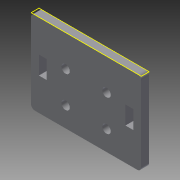
# Autodesk Inventor part: hook faceplate
Saved by Autodesk Inventor 2013 (Build 170138000, 138)
## iProperties
Created: 2013-01-26
Part Number: hook faceplate
Material: Generic
Document SubType Name: Modeling
Designer: Arpan
Density: 1 g/cm^3
Mass: 36.5886 g
Surface Area: 140.029 cm^2
Volume: 36.5886 cm^3
Author: Arpan
Autodesk Inventor part; units mm, degrees
ref_plane "YZ Plane" through (0, 0, 0) normal (1, 0, 0) x (0, 1, 0)
ref_plane "XZ Plane" through (0, 0, 0) normal (0, 1, 0) x (-1, 0, 0)
ref_plane "XY Plane" through (0, 0, 0) normal (0, 0, 1) x (1, 0, 0)
sketch "Sketch1" plane through (0, 0, 0) normal (0, 0, 1) x (1, 0, 0)
  line L0 (0, 0) -> (-88.9, 0)
  line L1 (-88.9, 0) -> (-88.9, 67.0052)
  line L2 (-88.9, 67.0052) -> (0, 67.0052)
  line L3 (0, 67.0052) -> (0, 0)
  dimension "d0" = 88.9
  dimension "d1" = 67.0052
  dimension "d2" = 90
  constraints: 8 end point, 2 perpendicular, 1 horizontal
  measures "d0" distance of L0.start L0.end
  measures "d1" distance of L0.end L1.end
  measures "d2" angle of L0 L3
extrude "Extrusion1" add sketch "Sketch1" along normal blind 6.35
sketch "Sketch2" plane through (-88.9, 67.0052, 0) normal (0, 1, 0) x (1, 0, 0)
  line L0 (0, 0) -> (88.9, 0) projected
  line L1 (0, 0) -> (0, -6.35) projected
  line L2 (88.9, -6.35) -> (0, -6.35) projected
  line L3 (88.9, 0) -> (88.9, -6.35) projected
sketch "Sketch3" plane through (0, 0, 0) normal (0, 0, -1) x (-1, 0, 0)
  line L0 (88.9, 0) -> (88.9, 67.0052) projected
  line L1 (0, 67.0052) -> (0, 0) projected
  line L2 (0, 67.0052) -> (0, 40.8178)
  line L3 (0, 40.8178) -> (6.35, 40.8178)
  line L4 (6.35, 40.8178) -> (6.35, 26.162)
  line L5 (6.35, 26.162) -> (12.7, 26.162)
  line L6 (12.7, 26.162) -> (12.7, 40.8178)
  line L7 (12.7, 40.8178) -> (6.35, 40.8178)
  line L8 (88.9, 40.8178) -> (82.55, 40.8178)
  line L9 (82.55, 40.8178) -> (82.55, 26.162)
  line L10 (82.55, 26.162) -> (76.2, 26.162)
  line L11 (76.2, 26.162) -> (76.2, 40.8178)
  line L12 (76.2, 40.8178) -> (82.55, 40.8178)
  dimension "d5" = 26.1874
  dimension "d6" = 6.35
  dimension "d7" = 14.6558
  dimension "d8" = 6.35
  dimension "d9" = 6.35
  dimension "d10" = 6.35
  dimension "d11" = 14.6558
  constraints: 22 end point, 4 parallel, 4 perpendicular, 2 collinear, 2 point on line
  measures "d5" distance of L1.start L2.end
  measures "d6" distance of L2.end L3.end
  measures "d7" distance of L3.end L4.end
  measures "d8" distance of L4.end L5.end
  measures "d9" distance of L8.start L8.end
  measures "d10" distance of L9.end L10.end
  measures "d11" distance of L10.end L11.end
extrude "Extrusion2" cut sketch "Sketch3" against normal blind 25.4
fillet "Fillet1" radius 3.175 4 edges at (0, 67.0052, 3.175) (0, 0, 3.175) (-88.9, 0, 3.175) (-88.9, 67.0052, 3.175)
sketch "Sketch4" plane through (0, 0, 0) normal (0, 0, -1) x (-1, 0, 0)
  circle A0 centre (60.96, 41.6) radius 3.3782 projected
  circle A1 centre (60.96, 16.2) radius 3.3782 projected
  circle A2 centre (27.94, 41.6) radius 3.3782 projected
  circle A3 centre (27.94, 16.2) radius 3.3782 projected
  point P0 (0, 0)
extrude "Extrusion3" cut sketch "Sketch4" against normal blind 25.4
body "Solid1"
